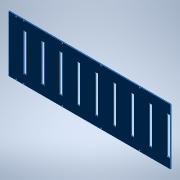
# Autodesk Inventor part: FerriteLayer
Saved by Autodesk Inventor 2021 (Build 250183000, 183)
## iProperties
Created: 2022-02-04
Part Number: FerriteLayer
Material: Generic
Document SubType Name: Modeling
Designer: tlar613
Density: 1 g/cm^3
Appearance: Default
Author: tlar613
Autodesk Inventor part; units mm, degrees
ref_plane "YZ Plane" through (0, 0, 0) normal (1, 0, 0) x (0, 1, 0)
ref_plane "XZ Plane" through (0, 0, 0) normal (0, 1, 0) x (-1, 0, 0)
ref_plane "XY Plane" through (0, 0, 0) normal (0, 0, 1) x (1, 0, 0)
sketch "Sketch1" plane through (0, 0, 0) normal (0, 0, 1) x (1, 0, 0)
  line L0 (-505, 165) -> (443.2, 165)
  line L1 (443.2, 165) -> (443.2, -165)
  line L2 (443.2, -165) -> (-505, -165)
  line L3 (-505, -165) -> (-505, 165)
  line L4 (0, 231) -> (0, -231) projected
  line L5 (-694.64, 0) -> (632.84, 0) projected
  line L6 (3.2, 108.4) -> (18, 108.4)
  line L7 (18, 108.4) -> (18, -108.4)
  line L8 (18, -108.4) -> (3.2, -108.4)
  line L9 (3.2, -108.4) -> (3.2, 108.4)
  line L10 (-101.8, 108.4) -> (-87, 108.4)
  line L11 (-87, 108.4) -> (-87, -108.4)
  line L12 (-87, -108.4) -> (-101.8, -108.4)
  line L13 (-101.8, -108.4) -> (-101.8, 108.4)
  line L14 (-206.8, 108.4) -> (-192, 108.4)
  line L15 (-192, 108.4) -> (-192, -108.4)
  line L16 (-192, -108.4) -> (-206.8, -108.4)
  line L17 (-206.8, -108.4) -> (-206.8, 108.4)
  line L18 (-311.8, 108.4) -> (-297, 108.4)
  line L19 (-297, 108.4) -> (-297, -108.4)
  line L20 (-297, -108.4) -> (-311.8, -108.4)
  line L21 (-311.8, -108.4) -> (-311.8, 108.4)
  line L22 (-416.8, 108.4) -> (-402, 108.4)
  line L23 (-402, 108.4) -> (-402, -108.4)
  line L24 (-402, -108.4) -> (-416.8, -108.4)
  line L25 (-416.8, -108.4) -> (-416.8, 108.4)
  line L26 (108.2, 108.4) -> (123, 108.4)
  line L27 (123, 108.4) -> (123, -108.4)
  line L28 (123, -108.4) -> (108.2, -108.4)
  line L29 (108.2, -108.4) -> (108.2, 108.4)
  line L30 (213.2, 108.4) -> (228, 108.4)
  line L31 (228, 108.4) -> (228, -108.4)
  line L32 (228, -108.4) -> (213.2, -108.4)
  line L33 (213.2, -108.4) -> (213.2, 108.4)
  line L34 (318.2, 108.4) -> (333, 108.4)
  line L35 (333, 108.4) -> (333, -108.4)
  line L36 (333, -108.4) -> (318.2, -108.4)
  line L37 (318.2, -108.4) -> (318.2, 108.4)
  line L38 (438, 108.4) -> (423.2, 108.4)
  line L39 (423.2, 108.4) -> (423.2, -108.4)
  line L40 (423.2, -108.4) -> (438, -108.4)
  line L41 (438, -108.4) -> (438, 108.4)
  line L42 (-505, 159) -> (443.2, 159) construction
  line L43 (-505, -159) -> (443.2, -159) construction
  circle A0 centre (-416.1, 159) radius 3
  circle A1 centre (-190.1, 159) radius 3
  circle A2 centre (35.9, 159) radius 3
  circle A3 centre (261.9, 159) radius 3
  circle A4 centre (-460.3, 159) radius 3
  circle A5 centre (-416.1, -159) radius 3
  circle A6 centre (-190.1, -159) radius 3
  circle A7 centre (261.9, -159) radius 3
  circle A8 centre (-460.3, -159) radius 3
  circle A9 centre (35.9, -159) radius 3
  point P0 (0, 0)
  dimension "d1" = 330
  dimension "d2" = 216.8
  dimension "d3" = 14.8
  dimension "d5" = 14.8
  dimension "d8" = 14.8
  dimension "d9" = 14.8
  dimension "d11" = 14.8
  dimension "d14" = 14.8
  dimension "d16" = 14.8
  dimension "d18" = 14.8
  dimension "d20" = 438
  dimension "d21" = 14.8
  dimension "d24" = 105
  dimension "d25" = 105
  dimension "d26" = 105
  dimension "d27" = 105
  dimension "d28" = 105
  dimension "d29" = 105
  dimension "d30" = 105
  dimension "d31" = 105
  dimension "d32" = 505
  dimension "d33" = 5.2
  dimension "d34" = 6
  dimension "d35" = 6
  dimension "d36" = 6
  dimension "d37" = 88.9
  dimension "d38" = 88.9
  dimension "d39" = 226
  dimension "d40" = 226
  dimension "d41" = 226
  dimension "d42" = 226
  dimension "d43" = 226
  dimension "d44" = 226
  dimension "d45" = 44.7
  dimension "d46" = 44.7
  constraints: 84 end point, 20 parallel, 15 collinear, 14 point on line, 11 horizontal, 11 perpendicular, 10 centre point, 9 equal radius, 3 other
  measures "d1" distance of L0.end L1.end
  measures "d2" distance of L6.end L7.end
  measures "d3" distance of L6.start L6.end
  measures "d5" distance of L11.end L12.end
  measures "d8" distance of L15.end L16.end
  measures "d9" distance of L19.end L20.end
  measures "d11" distance of L23.end L24.end
  measures "d14" distance of L27.end L28.end
  measures "d16" distance of L31.end L32.end
  measures "d18" distance of L35.end L36.end
  measures "d20" distance between parallel lines of L4 L41
  measures "d21" distance of L39.end L40.end
  measures "d24" distance between parallel lines of L39 L37
  measures "d25" distance between parallel lines of L37 L33
  measures "d26" distance between parallel lines of L33 L29
  measures "d27" distance between parallel lines of L29 L9
  measures "d28" distance between parallel lines of L9 L13
  measures "d29" distance between parallel lines of L13 L17
  measures "d30" distance between parallel lines of L17 L21
  measures "d31" distance between parallel lines of L21 L25
  measures "d32" distance between parallel lines of L3 L4
  measures "d33" distance between parallel lines of L1 L41
  measures "d34" distance between parallel lines of L0 L42
  measures "d35" distance between parallel lines of L2 L43
  measures "d36" diameter of A5
  measures "d37" distance from line of L3 A5.centre
  measures "d38" distance from line of A0.centre L3
  measures "d39" distance of A1.centre A0.centre
  measures "d40" distance of A2.centre A1.centre
  measures "d41" distance of A3.centre A2.centre
  measures "d42" distance of A6.centre A5.centre
  measures "d43" distance of A9.centre A6.centre
  measures "d44" distance of A7.centre A9.centre
  measures "d45" distance from line of L3 A4.centre
  measures "d46" distance from line of L3 A8.centre
extrude "Extrusion1" add sketch "Sketch1" along normal blind 5 contours L0 L4 L5 L11 L10 L13 L15 L14 L17 L19 L18 L21 L23 L22 L25 L3 | L0 L1 L5 L41 L38 L39 L35 L34 L37 L31 L30 L33 L27 L26 L29 L7 L6 L9 L4 | L5 L25 L24 L23 L21 L20 L19 L17 L16 L15 L13 L12 L11 L4 L2 L3 | L5 L9 L8 L7 L29 L28 L27 L33 L32 L31 L37 L36 L35 L39 L40 L41 L1 L2 L4
body "Solid1"
